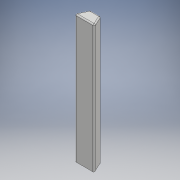
# Autodesk Inventor part: Tooth1
Saved by Autodesk Inventor 2018 (Build 220112000, 112)
## iProperties
Created: 2018-06-05
Part Number: Tooth1
Material: Generic
Document SubType Name: Modeling
Designer: P241310
Density: 1 g/cm^3
Appearance: Default
Author: P241310
Autodesk Inventor part; units mm, degrees
ref_plane "YZ Plane" through (0, 0, 0) normal (1, 0, 0) x (0, 1, 0)
ref_plane "XZ Plane" through (0, 0, 0) normal (0, 1, 0) x (-1, 0, 0)
ref_plane "XY Plane" through (0, 0, 0) normal (0, 0, 1) x (1, 0, 0)
sketch "Sketch1" plane through (0, 0, 0) normal (0, 0, 1) x (1, 0, 0)
  line L0 (0, 0) -> (2.56, 0)
  line L1 (2.56, 0) -> (2.56, 1.3618)
  line L2 (1.28, 0) -> (1.28, 4.701) construction
  line L3 (1.925, 1.3618) -> (2.56, 0)
  line L4 (0.635, 1.3618) -> (0, 0) construction
  line L5 (0.635, 1.3618) -> (1.925, 1.3618) construction
  line L6 (1.925, 1.3618) -> (2.56, 0) construction
  line L7 (0.635, 1.3618) -> (1.925, 1.3618)
  line L8 (0.635, 1.3618) -> (0, 0)
  dimension "d0" = 2.56
  dimension "d1" = 50
  dimension "d2" = 1.29
  constraints: 18 end point, 2 collinear, 1 horizontal, 1 midpoint, 1 parallel, 1 perpendicular, 1 point on line, 1 vertical
  measures "d0" distance of L0.start L0.end
  measures "d1" angle of L3 L4
  measures "d2" distance of L3.start L4.start
extrude "Extrusion1" add sketch "Sketch1" along normal blind 16
fillet "Fillet1" radius 0.15 11 edges at (0.635, 1.3618, 8) (1.925, 1.3618, 8) (1.28, 1.3618, 16) (1.28, 1.3618, 0) (1.28, 0, 16) (2.56, 0, 8) (0, 0, 8) (0.3175, 0.6809, 16) (2.2425, 0.6809, 16) (0.3175, 0.6809, 0) (2.2425, 0.6809, 0)
body "Solid1"
